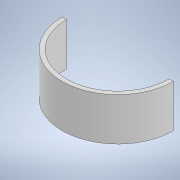
# Autodesk Inventor part: Pressure_seal
Saved by Autodesk Inventor 2022 (Build 260153000, 153)
## iProperties
Created: 2022-02-02
Part Number: Pressure_seal
Material: Generic
Document SubType Name: Modeling
Designer: Emazuddin Alif
Density: 1 g/cm^3
Appearance: Default
Author: Emazuddin Alif
Autodesk Inventor part; units mm, degrees
ref_plane "YZ Plane" through (0, 0, 0) normal (1, 0, 0) x (0, 1, 0)
ref_plane "XZ Plane" through (0, 0, 0) normal (0, 1, 0) x (-1, 0, 0)
ref_plane "XY Plane" through (0, 0, 0) normal (0, 0, 1) x (1, 0, 0)
sketch "Sketch1" plane through (0, 0, 0) normal (0, 1, 0) x (-1, 0, 0)
  arc A0 (15.24, 0) -> (-15.24, 0) centre (0, 0) ccw
  arc A1 (16.51, 0) -> (-16.51, 0) centre (0, 0) ccw
  line L0 (16.51, 0) -> (15.24, 0)
  line L1 (-16.51, 0) -> (-15.24, 0)
  dimension "d0" = 30.48
  dimension "d1" = 33.02
  constraints: 4 end point, 4 point on circle, 2 centre point, 2 coincident, 2 point on line, 1 horizontal
  measures "d0" diameter of A0
  measures "d1" diameter of A1
extrude "Extrusion1" add sketch "Sketch1" along normal blind 12.7
body "Solid1"
